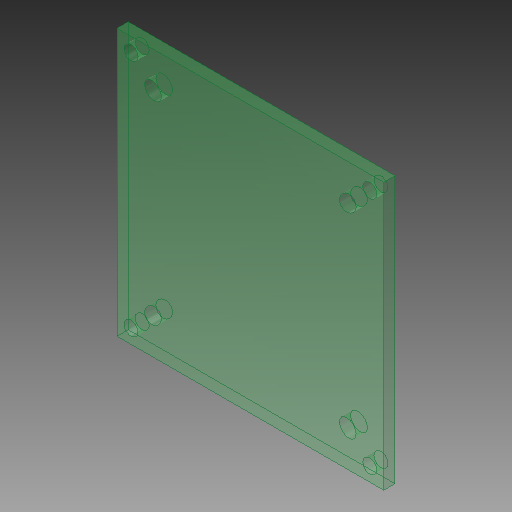
# Autodesk Inventor part: PCB_Camera
Saved by Autodesk Inventor 2017 (Build 210142000, 142)
## iProperties
Created: 2016-04-14
Part Number: PCB_Camera
Material: Generic
Document SubType Name: Modeling
Designer: Andres
Density: 1 g/cm^3
Appearance: Clear - Green 1
Mass: 2.26201 g
Surface Area: 31.588 cm^2
Volume: 2.26201 cm^3
Author: Andres
Autodesk Inventor part; units mm, degrees
ref_plane "YZ Plane" through (0, 0, 0) normal (1, 0, 0) x (0, 1, 0)
ref_plane "XZ Plane" through (0, 0, 0) normal (0, 1, 0) x (-1, 0, 0)
ref_plane "XY Plane" through (0, 0, 0) normal (0, 0, 1) x (1, 0, 0)
sketch "Sketch1" plane through (0, 0, 0) normal (0, 0, 1) x (1, 0, 0)
  line L0 (-19, 19) -> (19, 19)
  line L1 (19, 19) -> (19, -19)
  line L2 (19, -19) -> (-19, -19)
  line L3 (-19, -19) -> (-19, 19)
  point P0 (0, 0)
  point P1 (0, 19)
  point P2 (-19, 0)
  dimension "d0" = 38
  dimension "d1" = 38
  constraints: 8 end point, 2 midpoint, 2 parallel, 1 horizontal, 1 horizontal alignment, 1 perpendicular, 1 vertical alignment
  measures "d0" distance of L0.end L1.end
  measures "d1" distance of L1.end L2.end
extrude "Extrusion1" add sketch "Sketch1" along normal blind 1.6
sketch "Sketch2" plane through (0, 0, 1.6) normal (0, 0, 1) x (1, 0, 0)
  circle A0 centre (-17.006, 17.006) radius 1
  line L0 (19, 19) -> (-19, 19) projected
  line L1 (-19, 19) -> (-19, -19) projected
  line L2 (19, -19) -> (19, 19) projected
  line L3 (-19, -19) -> (19, -19) projected
  ellipse E0 centre (-13.876, 13.876) end of major axis (-12.9744, 12.9744) minor radius 1.1035
  line L4 (-19, 19) -> (19, -19)
  line L5 (0, 19) -> (0, -19)
  ellipse E1 centre (13.876, 13.876) end of major axis (12.9744, 12.9744) minor radius 1.1035
  line L6 (-19, 0) -> (19, 0)
  ellipse E2 centre (-13.876, -13.876) end of major axis (-12.9744, -12.9744) minor radius 1.1035
  ellipse E3 centre (13.876, -13.876) end of major axis (12.9744, -12.9744) minor radius 1.1035
  circle A1 centre (17.006, 17.006) radius 1
  circle A2 centre (-17.006, -17.006) radius 1
  circle A3 centre (17.006, -17.006) radius 1
  point P0 (0, 0)
  dimension "d52" = 1.1035
  dimension "d53" = 1.275
  dimension "d4" = 2
  dimension "d54" = 13.876
  dimension "d60" = 13.876
  dimension "d61" = 17.006
  dimension "d62" = 17.006
  constraints: 6 end point, 6 symmetric about line, 4 centre point, 4 midpoint, 2 horizontal, 1 vertical, 12 other
  measures "d4" diameter of A0
  measures "d54" horizontal distance of point (0, 0) point (-13.876, 13.876)
  measures "d60" horizontal distance of point (0, 0) point (-13.876, 13.876)
  measures "d61" horizontal distance of point (0, 0) A0.centre
  measures "d62" horizontal distance of point (0, 0) A0.centre
extrude "Extrusion3" cut sketch "Sketch2" against normal blind 1.6 contours A0 L4 | L4 A0 | L4 E0 | E0 L4 | E3 L4 | L4 E3 | A3 L4 | L4 A3 | E1 | E2 | A1 | A2
body "Solid1"
